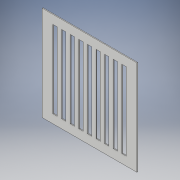
# Autodesk Inventor part: screen
Saved by Autodesk Inventor 2019 (Build 230136000, 136)
## iProperties
Created: 2018-07-11
Part Number: screen
Material: Generic
Document SubType Name: Modeling
Designer: User
Density: 1 g/cm^3
Appearance: Default
Author: User
Autodesk Inventor part; units mm, degrees
ref_plane "YZ Plane" through (0, 0, 0) normal (1, 0, 0) x (0, 1, 0)
ref_plane "XZ Plane" through (0, 0, 0) normal (0, 1, 0) x (-1, 0, 0)
ref_plane "XY Plane" through (0, 0, 0) normal (0, 0, 1) x (1, 0, 0)
sketch "Sketch1" plane through (0, 0, 0) normal (0, 0, 1) x (1, 0, 0)
  line L0 (-139.7, -139.7) -> (139.7, -139.7)
  line L1 (139.7, -139.7) -> (139.7, 139.7)
  line L2 (139.7, 139.7) -> (-139.7, 139.7)
  line L3 (-139.7, 139.7) -> (-139.7, -139.7)
  line L4 (-139.7, -139.7) -> (139.7, 139.7) construction
  line L5 (139.7, -139.7) -> (-139.7, 139.7) construction
  point P0 (0, 0)
  dimension "d0" = 279.4
  constraints: 12 end point, 2 midpoint, 2 parallel, 2 perpendicular, 1 horizontal
  measures "d0" distance of L1.end L2.end
extrude "Extrusion1" add sketch "Sketch1" along normal blind 2.54
sketch "Sketch3" plane through (0, 0, 2.54) normal (0, 0, 1) x (1, 0, 0)
  line L0 (-107.95, 114.3) -> (-95.25, 114.3)
  line L1 (-95.25, 114.3) -> (-95.25, -114.3)
  line L2 (-95.25, -114.3) -> (-107.95, -114.3)
  line L3 (-107.95, -114.3) -> (-107.95, 114.3)
  line L4 (-107.95, 114.3) -> (-95.25, -114.3) construction
  line L5 (-95.25, 114.3) -> (-107.95, -114.3) construction
  line L6 (0, 0) -> (-101.6, 0)
  line L7 (-139.7, 139.7) -> (-139.7, -139.7) projected
  line L8 (-139.7, -139.7) -> (139.7, -139.7) projected
  dimension "d11" = 12.7
  dimension "d12" = 31.75
  dimension "d13" = 25.4
  constraints: 14 end point, 2 horizontal, 2 midpoint, 2 parallel, 1 perpendicular
  measures "d11" distance of L1.end L2.end
  measures "d12" distance between parallel lines of L7 L3
  measures "d13" distance between parallel lines of L8 L2
extrude "Extrusion2" cut sketch "Sketch3" against normal up to next
pattern_linear "Rectangular Pattern1" count 9 spacing 25.4 along (1, 0, 0) of "Extrusion2"
body "Solid1"
